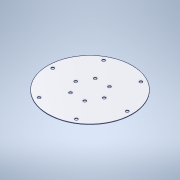
# Autodesk Inventor part: Filter
Saved by Autodesk Inventor 2020 (Build 240168000, 168)
## iProperties
Created: 2021-05-26
Part Number: Filter
Material: Generic
Document SubType Name: Modeling
Designer: Workshop
Density: 1 g/cm^3
Appearance: PTFE
Author: Workshop
Autodesk Inventor part; units mm, degrees
ref_plane "YZ Plane" through (0, 0, 0) normal (1, 0, 0) x (0, 1, 0)
ref_plane "XZ Plane" through (0, 0, 0) normal (0, 1, 0) x (-1, 0, 0)
ref_plane "XY Plane" through (0, 0, 0) normal (0, 0, 1) x (1, 0, 0)
sketch "Sketch1" plane through (0, 0, 0) normal (0, 0, 1) x (1, 0, 0)
  circle A0 centre (0, 0) radius 44 projected
  circle A1 centre (-14.925, 0) radius 1.5 projected
  circle A2 centre (-7.4625, 12.9254) radius 1.5 projected
  circle A3 centre (7.4625, 12.9254) radius 1.5 projected
  circle A4 centre (14.925, 0) radius 1.5 projected
  circle A5 centre (7.4625, -12.9254) radius 1.5 projected
  circle A6 centre (-7.4625, -12.9254) radius 1.5 projected
  circle A7 centre (-19.5, 33.775) radius 1.5 projected
  circle A8 centre (19.5, 33.775) radius 1.5 projected
  circle A9 centre (39, 0) radius 1.5 projected
  circle A10 centre (19.5, -33.775) radius 1.5 projected
  circle A11 centre (-19.5, -33.775) radius 1.5 projected
  circle A12 centre (-39, 0) radius 1.5 projected
extrude "Extrusion1" add sketch "Sketch1" along normal mid plane 0.5
body "Solid1"
